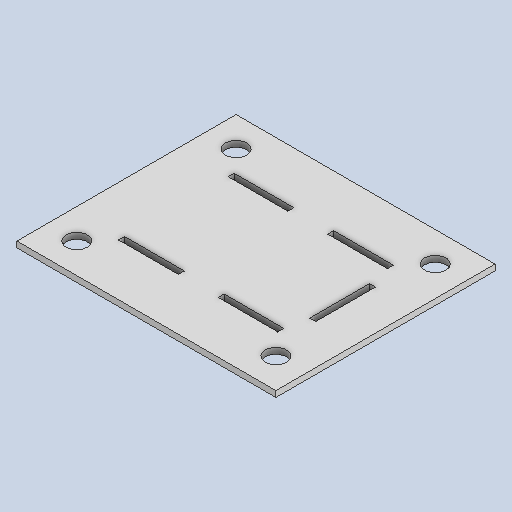
# Autodesk Inventor part: bottom_hinge_001
Saved by Autodesk Inventor 2025.2 (Build 292293000, 293)
## iProperties
Created: 2025-03-24
Part Number: bottom_hinge_001
Material: Generic
Document SubType Name: Sheet Metal
Designer: Caspe
Density: 1 g/cm^3
Sheet Metal Rule: Default_mm
Appearance: Default
Flat Pattern Width: 11 cm
Flat Pattern Length: 13 cm
Flat Pattern Area: 143 cm^2
Sheet Metal Width: 110,000 mm
Sheet Metal Length: 130,000 mm
Sheet Metal Area: 14300,000 mm^2
Author: Caspe
Autodesk Inventor part; units mm, degrees
ref_plane "YZ Plane" through (0, 0, 0) normal (1, 0, 0) x (0, 1, 0)
ref_plane "XZ Plane" through (0, 0, 0) normal (0, 1, 0) x (-1, 0, 0)
ref_plane "XY Plane" through (0, 0, 0) normal (0, 0, 1) x (1, 0, 0)
sketch "Sketch1" plane through (0, 0, 0) normal (0, 1, 0) x (-1, 0, 0)
  line L0 (0, 0) -> (-130, 0)
  line L1 (-130, 0) -> (-130, -110)
  line L2 (-130, -110) -> (0, -110)
  line L3 (0, -110) -> (0, 0)
  circle A0 centre (-15, -95) radius 5.35
  line L4 (-65, -110) -> (-65, 0)
  line L5 (0, -55) -> (-130, -55)
  circle A1 centre (-115, -95) radius 5.35
  circle A2 centre (-15, -15) radius 5.35
  circle A3 centre (-115, -15) radius 5.35
  dimension "d0" = 130
  dimension "d1" = 110
  dimension "d2" = 10.7
  dimension "d3" = 50
  dimension "d4" = 40
  measures "d0" distance of L2.end L1.end
  measures "d1" distance of L1.end L0.end
  measures "d2" diameter of A0
  measures "d3" distance from line of L4 A0.centre
  measures "d4" distance from line of L5 A0.centre
extrude "Plate1" add sketch "Sketch1" along normal blind 3
sketch "Sketch2" plane through (0, 3, 0) normal (0, 1, 0) x (1, 0, 0)
  line L0 (0, 110) -> (0, 0) projected
  line L1 (0, 55) -> (130, 55)
  line L2 (130, 0) -> (130, 110) projected
  line L3 (25, 84) -> (55, 84)
  line L4 (55, 84) -> (55, 81)
  line L5 (55, 81) -> (25, 81)
  line L6 (25, 81) -> (25, 84)
  line L7 (75, 81) -> (105, 81)
  line L8 (105, 81) -> (105, 84)
  line L9 (105, 84) -> (75, 84)
  line L10 (75, 84) -> (75, 81)
  line L11 (107, 55) -> (110, 55)
  line L12 (110, 55) -> (110, 70)
  line L13 (110, 70) -> (107, 70)
  line L14 (107, 70) -> (107, 55)
  line L15 (25, 26) -> (55, 26)
  line L16 (55, 26) -> (55, 29)
  line L17 (55, 29) -> (25, 29)
  line L18 (25, 29) -> (25, 26)
  line L19 (75, 29) -> (105, 29)
  line L20 (105, 29) -> (105, 26)
  line L21 (105, 26) -> (75, 26)
  line L22 (75, 26) -> (75, 29)
  line L23 (110, 55) -> (110, 40)
  line L24 (110, 40) -> (107, 40)
  line L25 (107, 40) -> (107, 55)
  point P0 (75, 82.5)
  point P1 (55, 82.5)
  dimension "d6" = 3
  dimension "d7" = 30
  dimension "d8" = 30
  dimension "d9" = 3
  dimension "d10" = 3
  dimension "d11" = 15
  dimension "d12" = 20
  dimension "d13" = 25
  dimension "d14" = 20
  dimension "d15" = 26
  constraints: 48 end point, 10 symmetric about line, 6 parallel, 4 midpoint, 3 horizontal, 3 perpendicular, 1 collinear, 1 point on line
  measures "d6" distance between parallel lines of L3 L5
  measures "d7" distance between parallel lines of L4 L6
  measures "d8" distance of L9.end L8.end
  measures "d9" distance of L8.end L7.end
  measures "d10" distance of L13.end L12.end
  measures "d11" distance between parallel lines of L1 L13
  measures "d12" distance of point (75, 82.5) point (55, 82.5)
  measures "d13" distance between parallel lines of L2 L8
  measures "d14" distance between parallel lines of L2 L12
  measures "d15" distance between parallel lines of L1 L7
extrude "Cut1" cut sketch "Sketch2" against normal blind 3
equation "\"d6\" = plate_thickness"
equation "\"d9\" = plate_thickness"
equation "\"d10\" = plate_thickness"
equation "\"d16\" = Thickness"
equation "\"d5\" = Thickness"
equation "\"Thickness\" = plate_thickness"
equation "\"BendRadius\" = Thickness"
equation "\"BendReliefWidth\" = Thickness"
equation "\"BendReliefDepth\" = 0.5 * Thickness"
equation "\"CornerReliefSize\" = 4 * Thickness"
equation "\"MinimumRemnant\" = 2 * Thickness"
equation "\"TransitionRadius\" = BendRadius"
equation "\"JacobiRadiusSize\" = BendRadius"
equation "\"GapSize\" = Thickness"
equation "\"A_width\" = 46"
equation "\"A_joint_diameter\" = 16"
equation "\"l___________\" = 0"
equation "\"l__________\" = 0"
equation "\"l_________\" = 0"
equation "\"rivet_diameter\" = 3.35"
equation "\"plate_thickness\" = 3"
equation "\"l________\" = 0"
equation "\"A_joint_tolerance\" = 3"
equation "\"A_B_spacing\" = 2"
equation "\"L_Piston_Bottom\" = 21"
equation "\"L_Piston_Top\" = 25"
equation "\"thin_plate\" = 1.5"
body "Solid1"
